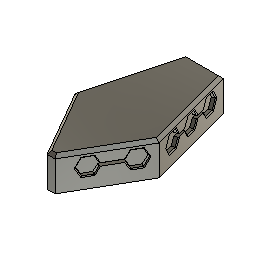
wedge_15deg_2mm (Autodesk Fusion 360 design; units mm, degrees)
Autodesk Fusion 360 part; units mm, degrees
sketch "case_bottom" plane through (0, 0, 0) normal (0, 0, 1) x (1, 0, 0)
  line L0 (-130.2878, -97.5223) -> (-16.5068, -128.0098)
  line L1 (-109.1239, -18.5374) -> (-130.2878, -97.5223)
  line L2 (-16.5068, -128.0098) -> (-3.6943, -109.7118)
  line L3 (-86.9858, -11.6525) -> (-109.1239, -18.5374)
  line L4 (-47.4404, -17.0197) -> (-47.5261, -16.9782)
  line L5 (-47.5261, -16.9782) -> (-66.0896, -12.0041)
  line L6 (-10.9673, -34.7188) -> (-47.4404, -17.0197)
  line L7 (-3.6943, -109.7118) -> (-22.3971, -77.3753)
  line L8 (-22.3971, -77.3753) -> (-10.9673, -34.7188)
  line L9 (-66.0896, -12.0041) -> (-86.9858, -11.6525)
  line L10 (-111.5937, -16.1638) -> (-133.962, -99.6436)
  line L11 (-133.962, -99.6436) -> (-15.2542, -131.4513)
  line L12 (-46.4735, -14.1544) -> (-65.6699, -9.0107)
  line L13 (-65.6699, -9.0107) -> (-87.4169, -8.6449)
  line L14 (-15.2542, -131.4513) -> (-0.1397, -109.8656)
  line L15 (-19.1773, -76.9502) -> (-7.4281, -33.1016)
  line L16 (-0.1397, -109.8656) -> (-19.1773, -76.9502)
  line L17 (-87.4169, -8.6449) -> (-111.5937, -16.1638)
  line L18 (-7.4281, -33.1016) -> (-46.4735, -14.1544)
  line L19 (-65.9217, -10.8067) -> (-87.1583, -10.4495)
  line L20 (-110.1118, -17.588) -> (-131.7575, -98.3709)
  line L21 (-9.5516, -34.0719) -> (-47.1051, -15.8486)
  line L22 (-16.0057, -129.3864) -> (-2.2725, -109.7733)
  line L23 (-47.1051, -15.8486) -> (-65.9217, -10.8067)
  line L24 (-87.1583, -10.4495) -> (-110.1118, -17.588)
  line L25 (-2.2725, -109.7733) -> (-21.1092, -77.2053)
  line L26 (-21.1092, -77.2053) -> (-9.5516, -34.0719)
  line L27 (-131.7575, -98.3709) -> (-16.0057, -129.3864)
  line L28 (-65.8378, -10.208) -> (-87.2445, -9.8479)
  line L29 (-132.4923, -98.7951) -> (-15.7552, -130.0747)
  line L30 (-110.6057, -17.1133) -> (-132.4923, -98.7951)
  line L31 (-46.6545, -15.4003) -> (-46.8946, -15.2839)
  line L32 (-1.5615, -109.8041) -> (-20.4652, -77.1202)
  line L33 (-20.4652, -77.1202) -> (-8.8438, -33.7485)
  line L34 (-15.7552, -130.0747) -> (-1.5615, -109.8041)
  line L35 (-46.8946, -15.2839) -> (-65.8378, -10.208)
  line L36 (-87.2445, -9.8479) -> (-110.6057, -17.1133)
  line L37 (-8.8438, -33.7485) -> (-46.6545, -15.4003)
  circle A0 centre (-88.6378, -32.8795) radius 2.2
  circle A1 centre (-98.4729, -69.5847) radius 2.2
  circle A2 centre (-38.4097, -46.3381) radius 2.2
  circle A3 centre (-34.1664, -92.8451) radius 2.2
  line L38 (-91.0167, -86.1903) -> (-122.8923, -77.6493)
  line L39 (-95.6755, -103.577) -> (-91.0167, -86.1903)
  line L40 (-127.551, -95.0359) -> (-95.6755, -103.577)
  line L41 (-122.8923, -77.6493) -> (-127.551, -95.0359)
  line L42 (-91.5925, -101.9586) -> (-93.1066, -107.6092)
  line L43 (-84.6064, -109.8868) -> (-83.0923, -104.2362)
  line L44 (-83.0923, -104.2362) -> (-91.5925, -101.9586)
  line L45 (-73.6279, -111.4154) -> (-72.7221, -108.0346)
  line L46 (-81.4154, -105.7053) -> (-82.3213, -109.086)
  line L47 (-82.3213, -109.086) -> (-73.6279, -111.4154)
  line L48 (-72.7221, -108.0346) -> (-81.4154, -105.7053)
  line L49 (-12.163, -97.5479) -> (-17.663, -88.0216)
  line L50 (-20.0438, -102.0979) -> (-12.163, -97.5479)
  line L51 (-25.5438, -92.5716) -> (-20.0438, -102.0979)
  line L52 (-17.663, -88.0216) -> (-25.5438, -92.5716)
  line L53 (-96.4921, -72.2377) -> (-98.7956, -80.8345)
  line L54 (-98.7956, -80.8345) -> (-90.4886, -83.0603)
  line L55 (-90.4886, -83.0603) -> (-88.1851, -74.4636)
  line L56 (-88.1851, -74.4636) -> (-96.4921, -72.2377)
  line L57 (1.8603, -131.9251) -> (1.8603, -9.9671)
  line L58 (88.327, -109.8868) -> (86.8129, -104.2362)
  line L59 (137.6826, -99.6436) -> (18.9748, -131.4513)
  line L60 (69.3905, -9.0107) -> (91.1375, -8.6449)
  line L61 (90.7065, -11.6525) -> (112.8445, -18.5374)
  line L62 (90.9651, -9.8479) -> (114.3264, -17.1133)
  line L63 (134.0084, -97.5223) -> (20.2274, -128.0098)
  line L64 (90.8789, -10.4495) -> (113.8324, -17.588)
  line L65 (29.2644, -92.5716) -> (23.7644, -102.0979)
  line L66 (86.8129, -104.2362) -> (95.3131, -101.9586)
  line L67 (21.3836, -88.0216) -> (29.2644, -92.5716)
  line L68 (131.2716, -95.0359) -> (99.3961, -103.577)
  line L69 (50.6152, -15.2839) -> (69.5584, -10.208)
  line L70 (15.8836, -97.5479) -> (21.3836, -88.0216)
  line L71 (91.1375, -8.6449) -> (115.3143, -16.1638)
  line L72 (18.9748, -131.4513) -> (3.8603, -109.8656)
  line L73 (14.6879, -34.7188) -> (51.161, -17.0197)
  line L74 (94.7373, -86.1903) -> (126.6129, -77.6493)
  line L75 (115.3143, -16.1638) -> (137.6826, -99.6436)
  line L76 (5.2822, -109.8041) -> (24.1859, -77.1202)
  line L77 (95.3131, -101.9586) -> (96.8272, -107.6092)
  line L78 (7.4149, -109.7118) -> (26.1177, -77.3753)
  line L79 (99.3961, -103.577) -> (94.7373, -86.1903)
  line L80 (77.3486, -111.4154) -> (76.4427, -108.0346)
  line L81 (69.8103, -12.0041) -> (90.7065, -11.6525)
  line L82 (113.8324, -17.588) -> (135.4781, -98.3709)
  line L83 (19.7263, -129.3864) -> (5.9931, -109.7733)
  line L84 (69.5584, -10.208) -> (90.9651, -9.8479)
  line L85 (91.9058, -74.4636) -> (100.2127, -72.2377)
  line L86 (11.1488, -33.1016) -> (50.1942, -14.1544)
  line L87 (114.3264, -17.1133) -> (136.213, -98.7951)
  line L88 (5.9931, -109.7733) -> (24.8298, -77.2053)
  circle A4 centre (42.1303, -46.3381) radius 2.2
  line L89 (102.5162, -80.8345) -> (94.2092, -83.0603)
  line L90 (85.136, -105.7053) -> (86.0419, -109.086)
  line L91 (69.6424, -10.8067) -> (90.8789, -10.4495)
  line L92 (50.3752, -15.4003) -> (50.6152, -15.2839)
  line L93 (50.1942, -14.1544) -> (69.3905, -9.0107)
  line L94 (22.898, -76.9502) -> (11.1488, -33.1016)
  line L95 (51.161, -17.0197) -> (51.2467, -16.9782)
  line L96 (94.2092, -83.0603) -> (91.9058, -74.4636)
  line L97 (13.2722, -34.0719) -> (50.8257, -15.8486)
  line L98 (112.8445, -18.5374) -> (134.0084, -97.5223)
  line L99 (100.2127, -72.2377) -> (102.5162, -80.8345)
  line L100 (19.4758, -130.0747) -> (5.2822, -109.8041)
  circle A5 centre (102.1935, -69.5847) radius 2.2
  line L101 (50.8257, -15.8486) -> (69.6424, -10.8067)
  circle A6 centre (37.887, -92.8451) radius 2.2
  line L102 (24.1859, -77.1202) -> (12.5644, -33.7485)
  line L103 (24.8298, -77.2053) -> (13.2722, -34.0719)
  line L104 (3.8603, -109.8656) -> (22.898, -76.9502)
  line L105 (136.213, -98.7951) -> (19.4758, -130.0747)
  line L106 (26.1177, -77.3753) -> (14.6879, -34.7188)
  line L107 (135.4781, -98.3709) -> (19.7263, -129.3864)
  line L108 (76.4427, -108.0346) -> (85.136, -105.7053)
  line L109 (12.5644, -33.7485) -> (50.3752, -15.4003)
  line L110 (86.0419, -109.086) -> (77.3486, -111.4154)
  line L111 (51.2467, -16.9782) -> (69.8103, -12.0041)
  line L112 (1.8603, -131.9251) -> (1.8603, -9.9671)
  circle A7 centre (92.3584, -32.8795) radius 2.2
  line L113 (126.6129, -77.6493) -> (131.2716, -95.0359)
  line L114 (23.7644, -102.0979) -> (15.8836, -97.5479)
  line L115 (20.2274, -128.0098) -> (7.4149, -109.7118)
  line L116 (-7.4281, -33.1016) -> (11.1488, -33.1016)
  line L117 (-0.1397, -109.8656) -> (3.8603, -109.8656)
  dimension "d6" = 2
  dimension "d7" = 2
  constraint vertical L57
  constraint horizontal L116
  constraint parallel L116 L117
  measures "d6" distance of L14.end L57
  measures "d7" distance of L72.end L112
extrude "Extrude2" add sketch "case_bottom" along normal blind 16.6 contours L15 L16 L57 L112 L116 L117 | L57 L94 L104 L112 L116 L117
sketch "Sketch7" plane through (2.1265, 0.5698, 0) normal (0.965926, 0.258819, 0) x (-0.258819, 0.965926, 0)
  line L0 (-80.2546, 0) -> (-34.8592, 0)
  line L1 (-34.8592, 0) -> (-34.8592, 16.6)
  line L2 (-34.8592, 16.6) -> (-80.2546, 16.6)
  line L3 (-80.2546, 16.6) -> (-80.2546, 0)
  line L4 (-80.2546, 9.7) -> (-34.8592, 9.7) construction
  line L5 (-68.2562, 13.6717) -> (-72.8461, 13.6783)
  line L6 (-72.8461, 13.6783) -> (-75.1468, 9.7067)
  line L7 (-75.1468, 9.7067) -> (-72.8576, 5.7283)
  line L8 (-72.8576, 5.7283) -> (-68.2677, 5.7217)
  line L9 (-68.2677, 5.7217) -> (-65.967, 9.6933)
  line L10 (-65.967, 9.6933) -> (-68.2562, 13.6717)
  line L11 (-55.2562, 13.6717) -> (-59.8461, 13.6783)
  line L12 (-59.8461, 13.6783) -> (-62.1468, 9.7067)
  line L13 (-62.1468, 9.7067) -> (-59.8576, 5.7283)
  line L14 (-59.8576, 5.7283) -> (-55.2677, 5.7217)
  line L15 (-55.2677, 5.7217) -> (-52.967, 9.6933)
  line L16 (-52.967, 9.6933) -> (-55.2562, 13.6717)
  line L17 (-42.2562, 13.6717) -> (-46.8461, 13.6783)
  line L18 (-46.8461, 13.6783) -> (-49.1468, 9.7067)
  line L19 (-49.1468, 9.7067) -> (-46.8576, 5.7283)
  line L20 (-46.8576, 5.7283) -> (-42.2677, 5.7217)
  line L21 (-42.2677, 5.7217) -> (-39.967, 9.6933)
  line L22 (-39.967, 9.6933) -> (-42.2562, 13.6717)
  line L23 (-70.5569, 8.95) -> (-44.5569, 8.95)
  arc A0 (-44.5569, 8.95) -> (-44.5569, 10.45) centre (-44.5569, 9.7) ccw
  line L24 (-44.5569, 10.45) -> (-70.5569, 10.45)
  arc A1 (-70.5569, 10.45) -> (-70.5569, 8.95) centre (-70.5569, 9.7) ccw
  line L25 (-70.5569, 9.7) -> (-44.5569, 9.7) construction
  point P0 (-57.5569, 9.7)
  point P1 (-70.5569, 9.7)
  point P2 (-44.5569, 9.7)
  point P3 (-70.5569, 9.7)
  point P4 (-57.5569, 9.7)
  point P5 (-44.5569, 9.7)
  dimension "d63" = 6.9
  dimension "d64" = 13
  dimension "d65" = 13
  dimension "d66" = 3.975
  dimension "d67" = 3.975
  dimension "d68" = 3.975
  dimension "d69" = 1.5
  constraint coincident L3 L4.start
  constraint coincident L1 L4.end
  constraint perpendicular L1 L4
  constraint coincident L4 P4
  constraint midpoint L4 P4
  constraint coincident L4 P3
  constraint coincident L4 P5
  constraint coincident P3 P1
  constraint coincident P4 P0
  constraint coincident P5 P2
  constraint tangent L23 A0
  constraint tangent A0 L24
  constraint parallel L23 L24
  constraint tangent L24 A1
  constraint tangent L23 A1
  constraint parallel L4 L25
  measures "d63" distance of L2 L4
  measures "d64" distance of P4 P3
  measures "d65" distance of P4 P5
  measures "d66" distance of P3 L10
  measures "d67" distance of P4 L16
  measures "d68" distance of P5 L22
  measures "d69" diameter of A0
sketch "Sketch9" plane through (50.5082, -29.213, 0) normal (0.865639, -0.500669, 0) x (0.500669, 0.865639, 0)
  line L0 (-93.1712, 0) -> (-55.1468, 0)
  line L1 (-55.1468, 0) -> (-55.1468, 16.6)
  line L2 (-55.1468, 16.6) -> (-93.1712, 16.6)
  line L3 (-93.1712, 16.6) -> (-93.1712, 0)
  line L4 (-93.1712, 9.7) -> (-55.1468, 9.7) construction
  line L5 (-55.1468, 16.6) -> (-55.1468, 0)
  line L6 (-78.8713, 13.6721) -> (-83.4612, 13.6778)
  line L7 (-83.4612, 13.6778) -> (-85.7611, 9.7057)
  line L8 (-85.7611, 9.7057) -> (-83.4711, 5.7279)
  line L9 (-83.4711, 5.7279) -> (-78.8811, 5.7222)
  line L10 (-78.8811, 5.7222) -> (-76.5812, 9.6943)
  line L11 (-76.5812, 9.6943) -> (-78.8713, 13.6721)
  line L12 (-60.8469, 13.6721) -> (-65.4368, 13.6778)
  line L13 (-65.4368, 13.6778) -> (-67.7367, 9.7057)
  line L14 (-67.7367, 9.7057) -> (-65.4467, 5.7279)
  line L15 (-65.4467, 5.7279) -> (-60.8567, 5.7222)
  line L16 (-60.8567, 5.7222) -> (-58.5568, 9.6943)
  line L17 (-58.5568, 9.6943) -> (-60.8469, 13.6721)
  line L18 (-81.1712, 8.95) -> (-63.1468, 8.95)
  arc A0 (-63.1468, 8.95) -> (-63.1468, 10.45) centre (-63.1468, 9.7) ccw
  line L19 (-63.1468, 10.45) -> (-81.1712, 10.45)
  arc A1 (-81.1712, 10.45) -> (-81.1712, 8.95) centre (-81.1712, 9.7) ccw
  line L20 (-81.1712, 9.7) -> (-63.1468, 9.7) construction
  point P0 (-81.1712, 9.7)
  point P1 (-63.1468, 9.7)
  point P2 (-81.1712, 9.7)
  point P3 (-63.1468, 9.7)
  dimension "d70" = 6.9
  dimension "d71" = 8
  dimension "d72" = 12
  dimension "d73" = 3.975
  dimension "d74" = 3.975
  dimension "d75" = 1.5
  constraint coincident L3 L4.start
  constraint coincident L1 L4.end
  constraint perpendicular L1 L4
  constraint coincident L4 P2
  constraint coincident L4 P3
  constraint coincident P2 P0
  constraint coincident P3 P1
  constraint tangent L18 A0
  constraint tangent A0 L19
  constraint parallel L18 L19
  constraint tangent L19 A1
  constraint tangent L18 A1
  constraint parallel L4 L20
  measures "d70" distance of L2 L4
  measures "d71" distance of P3 L5
  measures "d72" distance of L3 P2
  measures "d73" distance of P2 L11
  measures "d74" distance of P3 L17
  measures "d75" diameter of A0
sketch "Sketch11" plane through (-47.7203, -27.6005, 0) normal (-0.865639, -0.500669, 0) x (0.500669, -0.865639, 0)
  line L0 (57.0096, 0) -> (95.034, 0)
  line L1 (95.034, 0) -> (95.034, 16.6)
  line L2 (95.034, 16.6) -> (57.0096, 16.6)
  line L3 (57.0096, 16.6) -> (57.0096, 0)
  line L4 (57.0096, 9.7) -> (95.034, 9.7) construction
  line L5 (78.4441, 9.6781) -> (80.758, 5.7141)
  line L6 (80.758, 5.7141) -> (85.3479, 5.736)
  line L7 (85.3479, 5.736) -> (87.6239, 9.7219)
  line L8 (87.6239, 9.7219) -> (85.31, 13.6859)
  line L9 (85.31, 13.6859) -> (80.7201, 13.664)
  line L10 (80.7201, 13.664) -> (78.4441, 9.6781)
  line L11 (67.3235, 13.664) -> (62.7336, 13.6859)
  line L12 (62.7336, 13.6859) -> (60.4197, 9.7219)
  line L13 (60.4197, 9.7219) -> (62.6957, 5.736)
  line L14 (62.6957, 5.736) -> (67.2856, 5.7141)
  line L15 (67.2856, 5.7141) -> (69.5995, 9.6781)
  line L16 (69.5995, 9.6781) -> (67.3235, 13.664)
  line L17 (65.0096, 8.95) -> (83.034, 8.95)
  arc A0 (83.034, 8.95) -> (83.034, 10.45) centre (83.034, 9.7) ccw
  line L18 (83.034, 10.45) -> (65.0096, 10.45)
  arc A1 (65.0096, 10.45) -> (65.0096, 8.95) centre (65.0096, 9.7) ccw
  line L19 (65.0096, 9.7) -> (83.034, 9.7) construction
  point P0 (65.0096, 9.7)
  point P1 (83.034, 9.7)
  point P2 (83.034, 9.7)
  point P3 (65.0096, 9.7)
  dimension "d76" = 6.9
  dimension "d77" = 12
  dimension "d78" = 8
  dimension "d79" = 3.975
  dimension "d80" = 3.975
  dimension "d81" = 1.5
  constraint coincident L3 L4.start
  constraint coincident L1 L4.end
  constraint perpendicular L1 L4
  constraint coincident L4 P3
  constraint coincident L4 P2
  constraint coincident P2 P1
  constraint coincident P3 P0
  constraint tangent L17 A0
  constraint tangent A0 L18
  constraint parallel L17 L18
  constraint tangent L18 A1
  constraint tangent L17 A1
  constraint parallel L4 L19
  measures "d76" distance of L2 L4
  measures "d77" distance of L1 P2
  measures "d78" distance of L3 P3
  measures "d79" distance of P2 L10
  measures "d80" distance of P3 L16
  measures "d81" diameter of A0
sketch "Sketch12" plane through (1.3449, -0.3604, 0) normal (-0.965926, 0.258819, 0) x (-0.258819, -0.965926, 0)
  line L0 (33.8962, 0) -> (79.2916, 0)
  line L1 (79.2916, 0) -> (79.2916, 16.6)
  line L2 (79.2916, 16.6) -> (33.8962, 16.6)
  line L3 (33.8962, 16.6) -> (33.8962, 0)
  line L4 (33.8962, 9.7) -> (79.2916, 9.7) construction
  line L5 (45.8773, 13.6817) -> (41.2874, 13.6683)
  line L6 (41.2874, 13.6683) -> (39.004, 9.6866)
  line L7 (39.004, 9.6866) -> (41.3106, 5.7183)
  line L8 (41.3106, 5.7183) -> (45.9005, 5.7317)
  line L9 (45.9005, 5.7317) -> (48.1838, 9.7134)
  line L10 (48.1838, 9.7134) -> (45.8773, 13.6817)
  line L11 (58.8773, 13.6817) -> (54.2874, 13.6683)
  line L12 (54.2874, 13.6683) -> (52.004, 9.6866)
  line L13 (52.004, 9.6866) -> (54.3106, 5.7183)
  line L14 (54.3106, 5.7183) -> (58.9005, 5.7317)
  line L15 (58.9005, 5.7317) -> (61.1838, 9.7134)
  line L16 (61.1838, 9.7134) -> (58.8773, 13.6817)
  line L17 (71.8773, 13.6817) -> (67.2874, 13.6683)
  line L18 (67.2874, 13.6683) -> (65.004, 9.6866)
  line L19 (65.004, 9.6866) -> (67.3106, 5.7183)
  line L20 (67.3106, 5.7183) -> (71.9005, 5.7317)
  line L21 (71.9005, 5.7317) -> (74.1838, 9.7134)
  line L22 (74.1838, 9.7134) -> (71.8773, 13.6817)
  line L23 (43.5939, 8.95) -> (69.5939, 8.95)
  arc A0 (69.5939, 8.95) -> (69.5939, 10.45) centre (69.5939, 9.7) ccw
  line L24 (69.5939, 10.45) -> (43.5939, 10.45)
  arc A1 (43.5939, 10.45) -> (43.5939, 8.95) centre (43.5939, 9.7) ccw
  line L25 (43.5939, 9.7) -> (69.5939, 9.7) construction
  point P0 (43.5939, 9.7)
  point P1 (56.5939, 9.7)
  point P2 (69.5939, 9.7)
  point P3 (43.5939, 9.7)
  point P4 (56.5939, 9.7)
  point P5 (69.5939, 9.7)
  dimension "d82" = 6.9
  dimension "d83" = 13
  dimension "d84" = 13
  dimension "d85" = 3.975
  dimension "d86" = 3.975
  dimension "d87" = 3.975
  dimension "d88" = 1.5
  constraint coincident L3 L4.start
  constraint coincident L1 L4.end
  constraint perpendicular L1 L4
  constraint coincident L4 P3
  constraint midpoint L4 P4
  constraint coincident L4 P5
  constraint coincident P3 P0
  constraint coincident P4 P1
  constraint coincident P5 P2
  constraint tangent L23 A0
  constraint tangent A0 L24
  constraint parallel L23 L24
  constraint tangent L24 A1
  constraint tangent L23 A1
  constraint parallel L4 L25
  measures "d82" distance of L2 L4
  measures "d83" distance of P4 P5
  measures "d84" distance of P3 P4
  measures "d85" distance of P3 L10
  measures "d86" distance of P4 L16
  measures "d87" distance of P5 L22
  measures "d88" diameter of A0
extrude "Extrude11" cut sketch "Sketch9" against normal blind 2 contours L6 L7 L8 L9 L10 L11 L18 L19 A1 | L10 L11 L13 L14 L18 L19 | L10 L11 L18 L19 A1 | L13 L14 L18 A0 L19 | L12 L13 L14 L15 L16 L17 L18 A0 L19
extrude "Extrude12" cut sketch "Sketch7" against normal blind 2 contours L5 L6 L7 L8 L9 L10 L23 L24 A1 | L9 L10 L12 L13 L23 L24 | L9 L10 L23 L24 A1 | L12 L13 L15 L16 L23 L24 | L11 L12 L16 L24 | L15 L16 L18 L19 L23 L24 | L13 L14 L15 L23 | L18 L19 L23 A0 L24 | L17 L18 L19 L20 L21 L22 L23 A0 L24
extrude "Extrude13" cut sketch "Sketch12" against normal blind 2 contours L5 L6 L7 L8 L9 L10 L23 L24 A1 | L9 L10 L12 L13 L23 L24 | L9 L10 L23 L24 A1 | L12 L13 L15 L16 L23 L24 | L11 L12 L16 L24 | L15 L16 L18 L19 L23 L24 | L13 L14 L15 L23 | L18 L19 L23 A0 L24 | L17 L18 L19 L20 L21 L22 L23 A0 L24
extrude "Extrude14" cut sketch "Sketch11" against normal blind 2 contours L5 L10 L17 A0 L18 | L5 L10 L15 L16 L17 L18 | L5 L6 L7 L8 L9 L10 L17 A0 L18 | L15 L16 L17 L18 A1 | L11 L12 L13 L14 L15 L16 L17 L18 A1
chamfer "Chamfer2" distance 0.4 angle 45 60 edges at (-4.429, -102.4496, 11.7039) (-4.4195, -102.466, 7.7289) (-6.1382, -99.4943, 5.725) (-7.7601, -96.6902, 7.3321) (-6.1572, -99.4615, 13.675) (-7.7656, -96.6806, 12.057) (-13.5541, -86.6726, 12.057) (-15.1625, -83.8917, 13.675) (-16.8907, -80.9036, 11.7039) (-16.9002, -80.8872, 7.7289) (-15.1815, -83.8589, 5.725) (-13.5596, -86.663, 7.3321) (-17.5568, -70.9025, 11.6976) (-16.6644, -67.5717, 13.675) (-15.8316, -64.4636, 12.0591) (-15.8333, -64.4702, 7.3342) (-16.6704, -67.5942, 5.725) (-17.5599, -70.9137, 7.7226) (-14.1368, -58.1386, 12.0658) (-14.1385, -58.1452, 7.3409) (-13.3057, -55.0371, 5.725) (-12.4687, -51.9131, 7.3342) (-12.4669, -51.9066, 12.0591) (-13.2997, -55.0147, 13.675) (-10.7721, -45.5816, 12.0658) (-9.9351, -42.4576, 13.675) (-9.0456, -39.1381, 11.6774) (-9.0486, -39.1493, 7.7024) (-9.9411, -42.4801, 5.725) (-10.7739, -45.5882, 7.3409) (12.767, -39.1409, 11.6825) (13.6572, -42.4633, 13.675) (14.4932, -45.5833, 12.0642) (14.4941, -45.5865, 7.3392) (13.6602, -42.4744, 5.725) (12.7685, -39.1465, 7.7075) (16.188, -51.9082, 12.0608) (17.0219, -55.0203, 13.675) (17.8579, -58.1403, 12.0642) (17.8587, -58.1435, 7.3392) (17.0248, -55.0315, 5.725) (16.1889, -51.9115, 7.3358) (19.5526, -64.4653, 12.0608) (19.5535, -64.4685, 7.3358) (20.3895, -67.5885, 5.725) (21.2797, -70.9109, 7.7175) (21.2782, -70.9053, 11.6925) (20.3865, -67.5774, 13.675) (18.8951, -83.871, 13.675) (20.6174, -80.8932, 11.6832) (20.6149, -80.8975, 7.7082) (18.8901, -83.8796, 5.725) (17.2767, -86.6691, 7.3389) (17.2782, -86.6665, 12.0639) (11.4842, -96.6842, 12.0611) (9.8708, -99.4736, 13.675) (8.1461, -102.4557, 11.6918) (8.1436, -102.46, 7.7168) (9.8659, -99.4822, 5.725) (11.4827, -96.6867, 7.3361)
chamfer "Chamfer3" distance 1.5 angle 45 6 edges at (1.8603, -109.8656, 16.6) (13.3791, -93.4079, 16.6) (-9.6585, -93.4079, 16.6) (17.0234, -55.0259, 16.6) (-13.3027, -55.0259, 16.6) (1.8603, -33.1016, 16.6)
equation "rotation = 15 deg"
equation "mirror_offset = 2 mm"
equation "d6 = mirror_offset"
equation "d7 = mirror_offset"
